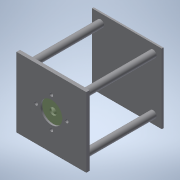
# Autodesk Inventor part: motor to gearbox flange
Saved by Autodesk Inventor 2020 (Build 240168000, 168)
## iProperties
Created: 2020-08-01
Part Number: motor to gearbox flange
Material: Generic
Document SubType Name: Modeling
Designer: Vikki
Density: 1 g/cm^3
Appearance: Default
Author: Vikki
Autodesk Inventor part; units mm, degrees
ref_plane "YZ Plane" through (0, 0, 0) normal (1, 0, 0) x (0, 1, 0)
ref_plane "XZ Plane" through (0, 0, 0) normal (0, 1, 0) x (-1, 0, 0)
ref_plane "Work Plane1" through (0, 0, 0) normal (0, 0, 1) x (1, 0, 0)
sketch "Sketch1" plane through (0, 0, 0) normal (0, 0, 1) x (1, 0, 0)
  line L0 (-40, -40) -> (40, -40)
  line L1 (40, -40) -> (40, 40)
  line L2 (40, 40) -> (-40, 40)
  line L3 (-40, 40) -> (-40, -40)
  line L4 (-40, -40) -> (40, 40) construction
  line L5 (40, -40) -> (-40, 40) construction
  point P0 (0, 0)
  dimension "d0" = 80
  constraints: 12 end point, 2 midpoint, 2 parallel, 2 perpendicular, 1 horizontal
  measures "d0" distance of L1.end L2.end
extrude "Extrusion1" add sketch "Sketch1" along normal blind 2
ref_plane "Work Plane2" through (-14.1414, -14.1414, 86.5) normal (0, 0, -1) x (0, 1, 0)
sketch "Sketch2" plane through (0, 0, 2) normal (0, 0, 1) x (1, 0, 0)
  circle A0 centre (0, 0) radius 42.5 construction
  circle A1 centre (30.052, 30.052) radius 4
  line L0 (0, 0) -> (30.052, 30.052) construction
  line L1 (-40, -40) -> (40, -40) projected
  circle A2 centre (-30.052, 30.052) radius 4
  circle A3 centre (-30.052, -30.052) radius 4
  circle A4 centre (30.052, -30.052) radius 4
  dimension "d3" = 85
  dimension "d4" = 45
  dimension "d5" = 8
  dimension "d8" = 360
  constraints: 4 centre point, 2 end point, 1 coincident, 12 other
  measures "d4" angle of L1 L0
  measures "d5" diameter of A1
extrude "Extrusion2" add sketch "Sketch2" along normal up to surface (84.5 mm away)
ref_plane "Work Plane3" through (0, 0, 86.5) normal (0, 0, -1) x (1, 0, 0)
sketch "Sketch3" plane through (0, 0, 86.5) normal (0, 0, -1) x (1, 0, 0)
  line L0 (40, -40) -> (-40, -40) projected
  circle A0 centre (30.052, -30.052) radius 4 projected
  circle A1 centre (-30.052, 30.052) radius 4 projected
  circle A2 centre (30.052, 30.052) radius 4 projected
  circle A3 centre (-30.052, -30.052) radius 4 projected
  line L1 (40, -40) -> (-40, -40) projected
  line L2 (-40, -40) -> (-40, 40) projected
  line L3 (-40, 40) -> (40, 40) projected
  line L4 (40, 40) -> (40, -40) projected
  circle A4 centre (0, 0) radius 12.5 projected
  circle A5 centre (-17.5, 0) radius 2 projected
  circle A6 centre (0, 17.5) radius 2 projected
  circle A7 centre (0, -17.5) radius 2 projected
  circle A8 centre (17.5, 0) radius 2 projected
  circle A9 centre (0, 0) radius 20.85 projected
  circle A10 centre (0, 0) radius 4 projected
  point P0 (0, 0)
  point P1 (40, -40)
  point P2 (-40, -40)
extrude "Extrusion3" add sketch "Sketch3" along normal blind 2 contours L0 L2 L3 L4 | A4 | A9
sketch "Sketch4" plane through (0, 0, 86.5) normal (0, 0, -1) x (1, 0, 0)
  line L0 (40, -40) -> (40, 40) projected
  line L1 (-40, -40) -> (40, -40) projected
  line L2 (-40, 40) -> (-40, -40) projected
  line L3 (40, 40) -> (-40, 40) projected
  circle A0 centre (0, 0) radius 12.5 projected
  line L4 (40, -40) -> (40, 40) projected
  line L5 (-40, -40) -> (40, -40) projected
  line L6 (-40, 40) -> (-40, -40) projected
  line L7 (40, 40) -> (-40, 40) projected
  circle A1 centre (0, 0) radius 4 projected
  circle A2 centre (0, 17.5) radius 2 projected
  circle A3 centre (0, -17.5) radius 2 projected
  circle A4 centre (-17.5, 0) radius 2 projected
  circle A5 centre (17.5, 0) radius 2 projected
  point P0 (0, 0)
extrude "Extrusion4" add sketch "Sketch4" against normal blind 2 contours L1 L2 L3 L0
body "Solid1"
